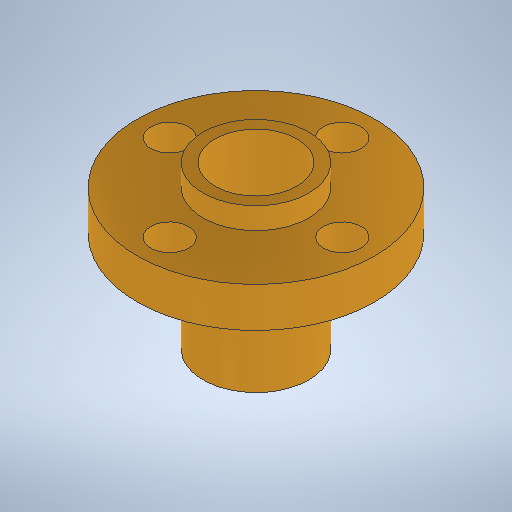
# Autodesk Inventor part: Lead nut
Saved by Autodesk Inventor 2025.2 (Build 292293000, 293)
## iProperties
Created: 2025-01-26
Part Number: Lead nut
Material: Generic
Document SubType Name: Modeling
Designer: caomi
Density: 1 g/cm^3
Appearance: Default
Author: caomi
Autodesk Inventor part; units mm, degrees
ref_plane "YZ Plane" through (0, 0, 0) normal (1, 0, 0) x (0, 1, 0)
ref_plane "XZ Plane" through (0, 0, 0) normal (0, 1, 0) x (-1, 0, 0)
ref_plane "XY Plane" through (0, 0, 0) normal (0, 0, 1) x (1, 0, 0)
sketch "Sketch1" plane through (0, 0, 0) normal (0, 0, 1) x (1, 0, 0)
  line L0 (3.8, 0) -> (3.8, 15)
  line L1 (3.8, 15) -> (4.9, 15)
  line L2 (4.9, 15) -> (4.9, 13)
  line L3 (4.9, 13) -> (11, 13)
  line L4 (11, 13) -> (11, 9.3)
  line L5 (11, 9.3) -> (4.9, 9.3)
  line L6 (4.9, 9.3) -> (4.9, 0)
  line L7 (4.9, 0) -> (3.8, 0)
  line L8 (-2.2, 0) -> (13.2, 0) projected
  line L9 (0, -3) -> (0, 18) projected
  point P0 (0, 0)
  point P1 (4.35, 0)
  point P2 (4.35, 15)
  point P3 (11, 11.15)
  dimension "d0" = 3.7
  dimension "d1" = 15
  dimension "d2" = 2
  dimension "d3" = 11
  dimension "d4" = 6.1
  dimension "d5" = 3.8
  constraints: 16 end point, 6 perpendicular, 3 midpoint, 3 point on line, 1 vertical
  measures "d0" distance between parallel lines of L3 L5
  measures "d1" distance from line of point (4.35, 0) L1
  measures "d2" distance from line of point (4.35, 15) L3
  measures "d3" horizontal distance of point (11, 11.15) point (0, 0)
  measures "d4" distance between parallel lines of L6 L4
  measures "d5" distance from line of L0 point (0, 0)
revolve "Revolution1" add sketch "Sketch1" angle 360 about axis through (0, -10, 0) along (0, 1, 0)
sketch "Sketch2" plane through (0, 13, 0) normal (0, 1, 0) x (1, 0, 0)
  circle A0 centre (0, 8) radius 1.75
  point P0 (0, 0)
  dimension "d7" = 3.5
  dimension "d8" = 8
  constraints: 1 centre point, 1 vertical alignment
  measures "d7" diameter of A0
  measures "d8" distance of A0.centre point (0, 0)
extrude "Extrusion1" cut sketch "Sketch2" against normal up to surface (3.7 mm away)
pattern_circular "Circular Pattern1" count 4 over 360 about axis through (0, 11.15, 0) along (0, 1, 0) of "Extrusion1"
body "Solid1"
